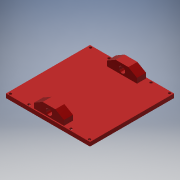
# Autodesk Inventor part: Gondola Top Frame
Saved by Autodesk Inventor 2018 (Build 220112000, 112)
## iProperties
Created: 2018-02-09
Part Number: Gondola Top Frame
Material: Steel, Alloy
Document SubType Name: Modeling
Designer: Joey
Density: 7.73 g/cm^3
Appearance: Smooth - Red
Author: Joey
Autodesk Inventor part; units mm, degrees
ref_plane "YZ Plane" through (0, 0, 0) normal (1, 0, 0) x (0, 1, 0)
ref_plane "XZ Plane" through (0, 0, 0) normal (0, 1, 0) x (-1, 0, 0)
ref_plane "XY Plane" through (0, 0, 0) normal (0, 0, 1) x (1, 0, 0)
sketch "Sketch1" plane through (0, 0, 0) normal (0, 0, 1) x (1, 0, 0)
  line L0 (-1066.8, 101.6) -> (1066.8, 101.6)
  line L1 (1066.8, 101.6) -> (1066.8, 0)
  line L2 (1066.8, 0) -> (-1066.8, 0)
  line L3 (-1066.8, 0) -> (-1066.8, 101.6)
  point P0 (0, 0)
  point P1 (0, 0)
  dimension "d0" = 2133.6
  dimension "d1" = 101.6
  constraints: 8 end point, 2 parallel, 1 coincident, 1 horizontal, 1 midpoint, 1 perpendicular
  measures "d0" distance of L0.start L0.end
  measures "d1" distance of L2.end L0.start
extrude "Extrusion1" add sketch "Sketch1" along normal mid plane 2133.6
sketch "Sketch2" plane through (-1066.8, 0, 1066.8) normal (0, -1, 0) x (1, 0, 0)
  line L0 (76.2, -76.2) -> (685.8, -76.2)
  line L1 (685.8, -76.2) -> (685.8, -2057.4)
  line L2 (685.8, -2057.4) -> (76.2, -2057.4)
  line L3 (76.2, -2057.4) -> (76.2, -76.2)
  line L4 (762, -76.2) -> (1371.6, -76.2)
  line L5 (1371.6, -76.2) -> (1371.6, -2057.4)
  line L6 (1371.6, -2057.4) -> (762, -2057.4)
  line L7 (762, -2057.4) -> (762, -76.2)
  line L8 (1447.8, -76.2) -> (2057.4, -76.2)
  line L9 (2057.4, -76.2) -> (2057.4, -2057.4)
  line L10 (2057.4, -2057.4) -> (1447.8, -2057.4)
  line L11 (1447.8, -2057.4) -> (1447.8, -76.2)
  line L12 (2133.6, 0) -> (2133.6, -2133.6) construction
  line L13 (0, 0) -> (2133.6, 0) construction
  line L14 (0, 0) -> (0, -2133.6) construction
  line L15 (2133.6, -2133.6) -> (0, -2133.6) construction
  line L16 (2133.6, 0) -> (0, 0) projected
  line L17 (1066.8, 0) -> (1066.8, -1066.8) construction
  line L18 (1066.8, -1066.8) -> (2133.6, -1066.8) construction
  line L19 (2133.6, 0) -> (2133.6, -2133.6) projected
  dimension "d4" = 76.2
  dimension "d5" = 76.2
  dimension "d6" = 76.2
  dimension "d7" = 76.2
  constraints: 28 end point, 6 parallel, 4 point on line, 3 horizontal, 3 perpendicular, 2 midpoint, 1 collinear, 1 vertical, 4 other
  measures "d4" distance between parallel lines of L7 L1
  measures "d5" distance between parallel lines of L11 L5
  measures "d6" distance between parallel lines of L14 L3
  measures "d7" distance between parallel lines of L4 L13
extrude "Extrusion2" cut sketch "Sketch2" against normal blind 76.2
sketch "Sketch3" plane through (-1066.8, 101.6, 1066.8) normal (0, 1, 0) x (1, 0, 0)
  line L0 (0, 2133.6) -> (2133.6, 2133.6) projected
  line L1 (0, 2133.6) -> (0, 0) projected
  circle A0 centre (63.5, 2082.8) radius 31.75
  circle A1 centre (63.5, 50.8) radius 31.75
  circle A2 centre (2070.1, 2082.8) radius 31.75
  circle A3 centre (2070.1, 50.8) radius 31.75
  circle A4 centre (533.4, 2082.8) radius 31.75
  circle A5 centre (533.4, 50.8) radius 31.75
  circle A6 centre (1600.2, 2082.8) radius 31.75
  circle A7 centre (1600.2, 50.8) radius 31.75
  point P0 (1066.8, 1066.8)
  dimension "d17" = 63.5
  dimension "d18" = 63.5
  dimension "d19" = 50.8
  dimension "d22" = 2032
  dimension "d25" = 2006.6
  dimension "d28" = 63.5
  dimension "d29" = 533.4
  dimension "d30" = 50.8
  dimension "d33" = 2032
  dimension "d36" = 1066.8
  constraints: 8 centre point, 2 horizontal, 2 vertical, 12 other
  measures "d17" diameter of A0
  measures "d18" distance from line of L1 A0.centre
  measures "d19" distance from line of L0 A0.centre
  measures "d22" distance of A0.centre A1.centre
  measures "d25" distance of A0.centre A2.centre
  measures "d28" diameter of A4
  measures "d29" distance from line of L1 A4.centre
  measures "d30" distance from line of L0 A4.centre
  measures "d33" distance of A4.centre A5.centre
  measures "d36" distance of A4.centre A6.centre
extrude "Extrusion3" cut sketch "Sketch3" against normal through all
sketch "Sketch4" plane through (0, 0, 0) normal (0, 0, 1) x (1, 0, 0)
  line L0 (1066.8, 101.6) -> (-1066.8, 101.6) projected
  line L1 (-381, 101.6) -> (-381, 228.6)
  line L2 (-381, 228.6) -> (-161.0295, 355.6)
  line L3 (-161.0295, 355.6) -> (161.0295, 355.6)
  line L4 (161.0295, 355.6) -> (381, 228.6)
  line L5 (381, 228.6) -> (381, 101.6)
  line L6 (0, 355.6) -> (0, 0) construction
  dimension "d42" = 127
  dimension "d43" = 254
  dimension "d50" = 762
  dimension "d60" = 150
  constraints: 12 end point, 2 point on line, 2 vertical, 1 midpoint, 1 parallel, 1 perpendicular, 2 other
  measures "d42" distance of L4.end L5.end
  measures "d43" distance between parallel lines of L0 L3
  measures "d50" distance between parallel lines of L5 L1
  measures "d60" angle of L3 L4
extrude "Extrusion4" add sketch "Sketch4" along normal mid plane 2082.8
sketch "Sketch5" plane through (381, 101.6, 1041.4) normal (1, 0, 0) x (0, 0, -1)
  line L0 (228.6, 254) -> (1854.2, 254)
  line L1 (1854.2, 254) -> (1854.2, 0)
  line L2 (1854.2, 0) -> (228.6, 0)
  line L3 (228.6, 0) -> (228.6, 254)
  line L4 (2082.8, 254) -> (0, 254) projected
  line L5 (1041.4, -101.6) -> (1041.4, -12.4327) construction
  line L6 (0, 0) -> (2082.8, 0) projected
  dimension "d47" = 1625.6
  constraints: 10 end point, 2 collinear, 2 parallel, 1 horizontal, 1 perpendicular, 1 vertical, 1 other
  measures "d47" distance between parallel lines of L1 L3
extrude "Extrusion5" cut sketch "Sketch5" against normal through all
sketch "Sketch6" plane through (0, 0, 1041.4) normal (0, 0, 1) x (1, 0, 0)
  line L0 (0, 0) -> (0, 215.9) construction
  line L1 (-203.2, 215.9) -> (203.2, 215.9) construction
  dimension "d51" = 203.2
  dimension "d52" = 215.9
  constraints: 4 end point, 1 horizontal, 1 midpoint, 1 symmetric about line, 1 vertical
  measures "d51" distance of L0.end L1.end
  measures "d52" distance of L0.start L0.end
hole "Hole1" at (0, 215.9, 1041.4) direction (0, 0, -1) diameter 159.7152 end through all
body "Solid1"
